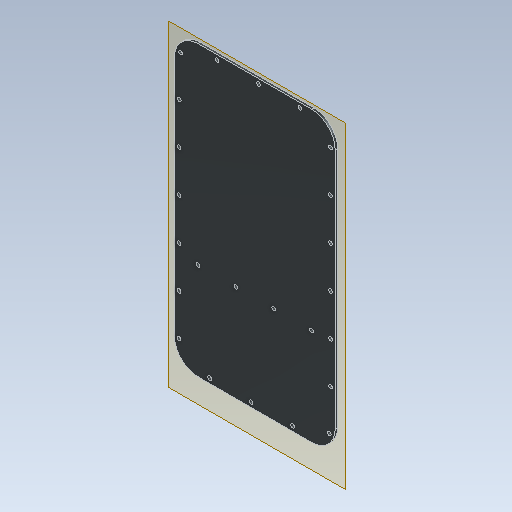
# Autodesk Inventor part: Крышка фонаря 2
Saved by Autodesk Inventor 2021 (Build 250183000, 183)
## iProperties
Created: 2020-12-11
Part Number: Крышка фонаря 2
Material: Чугун, серый
Document SubType Name: Modeling
Designer: Тимоха
Mass: 7294.7 g
Surface Area: 4201.82 cm^2
Volume: 1020.24 cm^3
Density: 7.15 g/cm^3
Appearance: Чугун серый
Author: Тимоха
Autodesk Inventor part; units mm, degrees
ref_plane "YZ Plane" through (0, 0, 0) normal (1, 0, 0) x (0, 1, 0)
ref_plane "XZ Plane" through (0, 0, 0) normal (0, 1, 0) x (-1, 0, 0)
ref_plane "XY Plane" through (0, 0, 0) normal (0, 0, 1) x (1, 0, 0)
ref_plane "РабПлоскость1" through (0, -25, 0) normal (0, 0, 1) x (1, 0, 0)
sketch "Эскиз1" plane through (0, -25, 0) normal (0, 0, 1) x (1, 0, 0)
  circle A0 centre (120, -75) radius 4 projected
  circle A1 centre (40, -75) radius 4 projected
  circle A2 centre (-40, -75) radius 4 projected
  circle A3 centre (-120, -75) radius 4 projected
  circle A4 centre (-95.2655, -270) radius 4 projected
  circle A5 centre (-7.6991, -270) radius 4 projected
  circle A6 centre (79.8673, -270) radius 4 projected
  circle A7 centre (157.0726, -245.0207) radius 4 projected
  circle A8 centre (160, -157.8319) radius 4 projected
  circle A9 centre (160, -70.2655) radius 4 projected
  circle A10 centre (160, 17.3009) radius 4 projected
  circle A11 centre (160, 104.8673) radius 4 projected
  circle A12 centre (160, 192.4336) radius 4 projected
  circle A13 centre (160, 280) radius 4 projected
  circle A14 centre (95.2655, 320) radius 4 projected
  circle A15 centre (7.6991, 320) radius 4 projected
  circle A16 centre (-79.8673, 320) radius 4 projected
  circle A17 centre (-157.0726, 295.0207) radius 4 projected
  circle A18 centre (-160, 207.8319) radius 4 projected
  circle A19 centre (-160, 120.2655) radius 4 projected
  circle A20 centre (-160, 32.6991) radius 4 projected
  circle A21 centre (-160, -54.8673) radius 4 projected
  circle A22 centre (-160, -142.4336) radius 4 projected
  circle A23 centre (-160, -230) radius 4 projected
  line L0 (170, -230) -> (170, 280) projected
  arc A24 (170, 280) -> (120, 330) centre (120, 280) ccw projected
  line L1 (120, 330) -> (-120, 330) projected
  arc A25 (-120, 330) -> (-170, 280) centre (-120, 280) ccw projected
  line L2 (-170, 280) -> (-170, -230) projected
  arc A26 (-170, -230) -> (-120, -280) centre (-120, -230) ccw projected
  line L3 (-120, -280) -> (120, -280) projected
  arc A27 (120, -280) -> (170, -230) centre (120, -230) ccw projected
  line L4 (-120, -95) -> (120, -95) projected
  arc A28 (150, -125) -> (120, -95) centre (120, -125) ccw projected
  line L5 (150, -125) -> (150, -230) projected
  arc A29 (120, -260) -> (150, -230) centre (120, -230) ccw projected
  line L6 (120, -260) -> (-120, -260) projected
  arc A30 (-150, -230) -> (-120, -260) centre (-120, -230) ccw projected
  line L7 (-150, -230) -> (-150, -125) projected
  arc A31 (-120, -95) -> (-150, -125) centre (-120, -125) ccw projected
  line L8 (150, 280) -> (150, -25) projected
  arc A32 (120, -55) -> (150, -25) centre (120, -25) ccw projected
  line L9 (120, -55) -> (-120, -55) projected
  arc A33 (-150, -25) -> (-120, -55) centre (-120, -25) ccw projected
  line L10 (-150, -25) -> (-150, 280) projected
  arc A34 (-120, 310) -> (-150, 280) centre (-120, 280) ccw projected
  line L11 (-120, 310) -> (120, 310) projected
  arc A35 (150, 280) -> (120, 310) centre (120, 280) ccw projected
  point P0 (0, 25)
extrude "Выдавливание1" add sketch "Эскиз1" along normal blind 5 contours A27 L3 A26 L2 A25 L1 A24 L0 | L4 A28 L5 A29 L6 A30 L7 A31 | L8 A32 L9 A33 L10 A34 L11 A35
